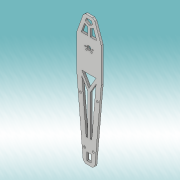
# Autodesk Inventor part: Leg_part3
Saved by Autodesk Inventor 2019 (Build 230136000, 136)
## iProperties
Created: 2019-01-31
Part Number: Leg_part3
Material: Generic
Document SubType Name: Modeling
Designer: USUARIO
Density: 1 g/cm^3
Appearance: Default
Author: USUARIO
Autodesk Inventor part; units mm, degrees
ref_plane "YZ Plane" through (0, 0, 0) normal (1, 0, 0) x (0, 1, 0)
ref_plane "XZ Plane" through (0, 0, 0) normal (0, 1, 0) x (-1, 0, 0)
ref_plane "XY Plane" through (0, 0, 0) normal (0, 0, 1) x (1, 0, 0)
sketch "Sketch1" plane through (0, 0, 0) normal (0, 0, 1) x (1, 0, 0)
  line L0 (0, 0) -> (-7, 0)
  line L1 (-7, 0) -> (-11.5963, 3.8567)
  line L2 (-11.5963, 3.8567) -> (-24, 148.3252)
  line L3 (-24, 148.3252) -> (-24, 216.3252)
  line L4 (-24, 216.3252) -> (-11.5963, 251.1842)
  line L5 (-11.5963, 251.1842) -> (-7, 255.0409)
  line L6 (-7, 255.0409) -> (0, 255.0409)
  line L7 (0, 255.0409) -> (0, 0)
  line L8 (0, 6) -> (-4, 6)
  line L9 (-4, 6) -> (-4, 21)
  line L10 (-4, 21) -> (0, 21)
  line L11 (-5.5, 46) -> (-2.5, 46)
  line L12 (-2.5, 46) -> (-2.5, 125.6208)
  line L13 (-2.5, 125.6208) -> (-14.0543, 145.6334)
  line L14 (-14.0543, 145.6334) -> (-5.5, 46)
  line L15 (0, 249.0409) -> (-5, 249.0409)
  line L16 (-5, 249.0409) -> (-7.135, 243.0409)
  line L17 (-7.135, 243.0409) -> (0, 238.9899)
  line L18 (-8.7779, 238.224) -> (-2.5, 234.6596)
  line L19 (-2.5, 234.6596) -> (-2.5, 220.224)
  line L20 (-2.5, 220.224) -> (-15.1828, 220.224)
  line L21 (-15.1828, 220.224) -> (-8.7779, 238.224)
  line L22 (0, 131.2907) -> (-14, 155.5394)
  line L23 (-14, 155.5394) -> (0, 155.5394)
  arc A0 (0, 204) -> (0, 196) centre (0, 200) ccw
  circle A1 centre (-7, 200) radius 1.5
  line L24 (0, 0) -> (7, 0)
  line L25 (7, 0) -> (11.5963, 3.8567)
  line L26 (11.5963, 3.8567) -> (24, 148.3252)
  line L27 (24, 148.3252) -> (24, 216.3252)
  line L28 (24, 216.3252) -> (11.5963, 251.1842)
  line L29 (11.5963, 251.1842) -> (7, 255.0409)
  line L30 (7, 255.0409) -> (0, 255.0409)
  line L31 (0, 6) -> (4, 6)
  line L32 (4, 6) -> (4, 21)
  line L33 (4, 21) -> (0, 21)
  line L34 (5.5, 46) -> (2.5, 46)
  line L35 (2.5, 46) -> (2.5, 125.6208)
  line L36 (2.5, 125.6208) -> (14.0543, 145.6334)
  line L37 (14.0543, 145.6334) -> (5.5, 46)
  line L38 (0, 249.0409) -> (5, 249.0409)
  line L39 (5, 249.0409) -> (7.135, 243.0409)
  line L40 (7.135, 243.0409) -> (0, 238.9899)
  line L41 (8.7779, 238.224) -> (2.5, 234.6596)
  line L42 (2.5, 234.6596) -> (2.5, 220.224)
  line L43 (2.5, 220.224) -> (15.1828, 220.224)
  line L44 (15.1828, 220.224) -> (8.7779, 238.224)
  line L45 (0, 131.2907) -> (14, 155.5394)
  line L46 (14, 155.5394) -> (0, 155.5394)
  arc A2 (0, 196) -> (0, 204) centre (0, 200) ccw
  circle A3 centre (-16.5993, 116.8252) radius 2
  circle A4 centre (16.5993, 116.8252) radius 2
  circle A5 centre (-8.5, 27) radius 2
  circle A6 centre (8.5, 27) radius 2
  line L47 (0, 200) -> (-10, 200)
  line L48 (0, 204) -> (-14, 204)
  line L49 (0, 196) -> (-14, 196)
  circle A7 centre (-4.9497, 195.0503) radius 1.5
  circle A8 centre (0, 193) radius 1.5
  circle A9 centre (4.9497, 195.0503) radius 1.5
  circle A10 centre (7, 200) radius 1.5
  circle A11 centre (0, 207) radius 1.5
  dimension "d0" = 7
  dimension "d1" = 6
  dimension "d2" = 145
  dimension "d3" = 68
  dimension "d4" = 37
  dimension "d5" = 48
  dimension "d8" = 140
  dimension "d9" = 140
  dimension "d10" = 15
  dimension "d11" = 6
  dimension "d12" = 4
  dimension "d13" = 3
  dimension "d14" = 5
  dimension "d15" = 25
  dimension "d17" = 100
  dimension "d19" = 5
  dimension "d20" = 28
  dimension "d21" = 150
  dimension "d29" = 6
  dimension "d32" = 6
  dimension "d33" = 4
  dimension "d38" = 3
  dimension "d42" = 4
  dimension "d43" = 31.5
  dimension "d45" = 5
  dimension "d46" = 4
  dimension "d47" = 17
  dimension "d48" = 6
  dimension "d51" = 200
  dimension "d54" = 3
  dimension "d56" = 14
  dimension "d57" = 8
  dimension "d58" = 7
  dimension "d61" = 180
  dimension "d63" = 5
  dimension "d64" = 5
  dimension "d65" = 100
  dimension "d66" = 7
  dimension "d67" = 5
  dimension "d68" = 18
  constraints: 98 end point, 21 horizontal alignment, 12 centre point, 10 horizontal, 5 parallel, 5 perpendicular, 4 point on circle, 2 coincident, 2 equal length, 2 equal radius, 1 concentric, 1 symmetric about line, 22 other
  measures "d0" distance of L0.start L0.end
  measures "d1" distance of L0.end L1.end
  measures "d2" distance of L1.end L2.end
  measures "d3" distance of L2.end L3.end
  measures "d4" distance of L3.end L4.end
  measures "d8" angle of L0 L1
  measures "d9" angle of L6 L5
  measures "d10" distance of L8.end L9.end
  measures "d11" distance between parallel lines of L0 L8
  measures "d12" distance of L9.end L10.end
  measures "d13" distance of L11.start L11.end
  measures "d15" distance between parallel lines of L10 L11
  measures "d17" distance of L13.end L11.start
  measures "d19" distance between parallel lines of L22 L13
  measures "d20" distance of L22.start L22.end
  measures "d21" angle of L13 L12
  measures "d29" distance between parallel lines of L6 L15
  measures "d32" vertical distance of L15.end L16.end
  measures "d33" radius of A0
  measures "d38" diameter of A1
  measures "d42" diameter of A3
  measures "d43" vertical distance of L2.end A3.centre
  measures "d45" distance from line of L14 A3.centre
  measures "d46" diameter of A5
  measures "d48" distance from line of L10 A5.centre
  measures "d51" distance from line of L24 A0.centre
  measures "d54" distance of L47.end A1.centre
  measures "d56" distance of L48.start L48.end
  measures "d57" diameter of A1.centre L48
  measures "d58" distance of A0.centre A1.centre
  measures "d64" distance between parallel lines of L17 L18
  measures "d65" angle of L17 L16
  measures "d66" distance between parallel lines of L21 L4
  measures "d67" distance of L15.start L15.end
  measures "d68" distance from line of L18.start L20
extrude "Extrusion1" add sketch "Sketch1" along normal mid plane 4 contours L0 L1 L2 L3 L4 L5 L6 L7 L15 L16 L17 A11 A0 A8 L23 L22 L10 L9 L8 | L7 L31 L32 L33 L45 L46 A8 A2 A11 L40 L39 L38 L30 L29 L28 L27 L26 L25 L24 | A8 L7 | L7 A8 | A11 L7 | L7 A11
body "Solid1"
